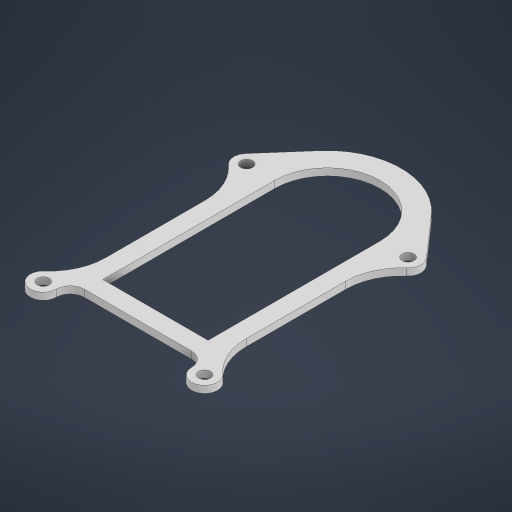
# Autodesk Inventor part: Skirt
Saved by Autodesk Inventor 2023 (Build 270158000, 158)
## iProperties
Created: 2022-10-14
Part Number: Skirt
Material: 一般
Document SubType Name: Modeling
Designer: hide
Density: 1 g/cm^3
Appearance: 既定
Author: hide
Autodesk Inventor part; units mm, degrees
ref_plane "YZ Plane" through (0, 0, 0) normal (1, 0, 0) x (0, 1, 0)
ref_plane "XZ Plane" through (0, 0, 0) normal (0, 1, 0) x (-1, 0, 0)
ref_plane "XY Plane" through (0, 0, 0) normal (0, 0, 1) x (1, 0, 0)
sketch "スケッチ1" plane through (0, 0, 0) normal (0, 1, 0) x (-1, 0, 0)
  circle A0 centre (11.5, 0) radius 0.85
  circle A1 centre (11.5, 29) radius 0.85
  line L0 (0, -11.6446) -> (0, 36.0381)
  arc A2 (12.7208, 27.61) -> (9.65, 29) centre (11.5, 29) ccw
  arc A3 (12.8915, -1.2191) -> (12.7208, 1.39) centre (11.5, 0) ccw
  circle A4 centre (0, 0) radius 7.5
  line L1 (7.5, 24.5) -> (7.5, 0)
  line L2 (7.5, 0) -> (2.3298, -4.6119)
  line L3 (12.8915, -1.2191) -> (7.8978, -6.9191)
  arc A5 (0, -10.5) -> (7.8978, -6.9191) centre (0, 0) ccw
  circle A6 centre (0, -2) radius 3.5
  line L4 (7.5, 24.5) -> (0, 24.5)
  line L5 (14.3325, 28.15) -> (9.1092, 28.15)
  line L6 (-7.5, 24.5) -> (-7.5, 0)
  line L7 (-7.5, 0) -> (-2.3298, -4.6119)
  line L8 (-7.5, 24.5) -> (0, 24.5)
  line L9 (10, 7.4008) -> (10, 21.5992)
  arc A7 (7.65, 27) -> (9.65, 29) centre (7.65, 29) ccw
  line L10 (7.65, 27) -> (0, 27)
  arc A8 (12.7208, 27.61) -> (10, 21.5992) centre (18, 21.5992) ccw
  arc A9 (10, 7.4008) -> (12.7208, 1.39) centre (18, 7.4008) ccw
  point P0 (0, 30.9357)
  point P1 (0, 26.85)
  point P2 (7.4841, 0.4881)
  point P3 (0, 26.5)
  point P4 (0, -5.5)
  point P5 (-2.3298, -4.6119)
  point P6 (0, 1.5)
  point P7 (-7.5, 0)
  point P8 (0, -7.5)
  dimension "d7" = 15
  dimension "d23" = 7
  dimension "d2" = 29
  dimension "d10" = 1
  dimension "d11" = 1
  dimension "d18" = 10.5
  dimension "d24" = 1.7
  dimension "d25" = 2
  dimension "d39" = 15
  dimension "d41" = 2.5
  dimension "d43" = 2.5
  dimension "d44" = 8
  dimension "d45" = 23
  dimension "d47" = 2
  constraints: 20 end point, 12 point on circle, 9 tangent, 8 centre point, 5 horizontal alignment, 4 coincident, 2 equal radius, 2 horizontal, 1 vertical, 1 vertical alignment, 18 other
  measures "d2" distance of A1.centre A0.centre
  measures "d10" radial gap between concentric circles of A3 A0
  measures "d11" radial gap between concentric circles of A2 A1
  measures "d18" radius of A5
  measures "d24" diameter of A0
  measures "d25" distance of point (0, 0) point (0, -2)
  measures "d41" distance between parallel lines of L10 L4
  measures "d43" distance between parallel lines of L9 L1
  measures "d44" radius of A9
  measures "d47" radius of A7
extrude "押し出し1" add sketch "スケッチ1" along normal blind 1 contours L5 A7 A2 | L5 A2 A8 L9 A9 A3 L3 A5 L0 A4 L1 L4 L10 A7
mirror "ミラー1" about plane through (0, 0, 0) normal (1, 0, 0) of "押し出し1"
